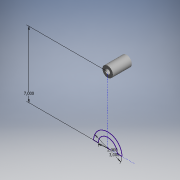
# Autodesk Inventor part: Biela
Saved by Autodesk Inventor 2019.3 (Build 233278000, 278)
## iProperties
Part Number: Biela
Material: Generic
Document SubType Name: Modeling
Designer: Usuario
Appearance: Default
Author: Usuario
Autodesk Inventor part; units mm, degrees
ref_plane "YZ Plane" through (0, 0, 0) normal (1, 0, 0) x (0, 1, 0)
ref_plane "XZ Plane" through (0, 0, 0) normal (0, 1, 0) x (-1, 0, 0)
ref_plane "XY Plane" through (0, 0, 0) normal (0, 0, 1) x (1, 0, 0)
sketch "Sketch1" plane through (0, 0, 0) normal (0, 0, 1) x (1, 0, 0)
  circle A0 centre (0, 0) radius 6.35
  circle A1 centre (0, 0) radius 13.97
  dimension "d0" = 12.7
  dimension "d1" = 27.94
  constraints: 2 centre point, 2 coincident
  measures "d0" diameter of A0
  measures "d1" diameter of A1
extrude "Extrusion1" add sketch "Sketch1" along normal blind 50.8
sketch "Sketch2" plane through (0, 0, 50.8) normal (0, 0, 1) x (1, 0, 0)
  line L0 (0, 0) -> (0, -177.8) construction
  arc A0 (25.4, -177.8) -> (-25.4, -177.8) centre (0, -177.8) ccw
  arc A1 (38.1, -177.8) -> (-38.1, -177.8) centre (0, -177.8) ccw
  line L1 (0, -177.8) -> (-93.8038, -177.8) construction
  line L2 (0, -177.8) -> (9.382, -177.8)
  line L3 (9.382, -177.8) -> (72.78, -177.8) construction
  line L4 (-38.1, -177.8) -> (-25.4, -177.8) construction
  line L5 (-38.1, -177.8) -> (-25.4, -177.8)
  line L6 (25.4, -177.8) -> (38.1, -177.8)
  dimension "d5" = 50.8
  dimension "d6" = 76.2
  dimension "d7" = 177.8
  constraints: 14 end point, 5 point on line, 4 point on circle, 2 centre point, 2 coincident, 2 collinear, 2 horizontal, 1 vertical
  measures "d5" diameter of A0
  measures "d6" diameter of A1
  measures "d7" distance of L0.end L0.start
body "Solid1"
